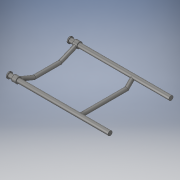
# Autodesk Inventor part: front bar
Saved by Autodesk Inventor 2018 (Build 220112000, 112)
## iProperties
Created: 2018-01-14
Part Number: front bar
Material: Aluminum 6061
Document SubType Name: Modeling
Designer: prakh
Density: 2.7 g/cm^3
Appearance: Anodized - Light Gray
Author: prakh
Autodesk Inventor part; units mm, degrees
ref_plane "XZ Plane" through (0, 0, 0) normal (0, 1, 0) x (-1, 0, 0)
ref_plane "XY Plane" through (0, 0, 0) normal (0, 0, 1) x (1, 0, 0)
sketch "Sketch1" plane through (0, 0, 0) normal (0, 0, 1) x (1, 0, 0)
  circle A0 centre (0, 0) radius 12.7
  dimension "d0" = 25.4
  constraints: 1 centre point, 1 coincident
  measures "d0" diameter of A0
sketch "Sketch2" plane through (0, 0, 0) normal (1, 0, 0) x (0, 1, 0)
  line L0 (0, 88.9) -> (0, -88.9)
  line L1 (0, -88.9) -> (48.2558, -206.375)
  line L2 (0, 88.9) -> (48.2558, 206.375)
  line L3 (48.2558, -206.375) -> (232.1871, -206.375) construction
  point P0 (0, 0)
  dimension "d1" = 88.9
  dimension "d2" = 177.8
  dimension "d3" = 412.75
  dimension "d5" = 127
  dimension "d26" = 112.332
  constraints: 8 end point, 2 vertical alignment, 1 equal length, 1 horizontal, 1 vertical
  measures "d1" distance of point (0, 0) L0.end
  measures "d2" distance of L0.start L0.end
  measures "d3" distance of L1.end L2.end
  measures "d5" distance of L0.start L2.end
  measures "d26" angle of L1 L3
sweep "Sweep1" add profiles "Sketch1" path "Sketch2"
ref_plane "Work Plane1" through (381, 0, 0) normal (1, 0, 0) x (0, 1, 0)
sketch "Sketch3" plane through (0, 0, 0) normal (0, 0, 1) x (1, 0, 0)
  circle A0 centre (381, 0) radius 12.7
  point P0 (0, 0)
  dimension "d9" = 381
  dimension "d10" = 25.4
  constraints: 1 centre point
  measures "d9" distance of point (0, 0) A0.centre
  measures "d10" diameter of A0
sketch "Sketch4" plane through (381, 0, 0) normal (1, 0, 0) x (0, 1, 0)
  line L0 (60.0033, 201.5494) -> (36.5083, 211.2006) projected
  line L1 (48.2558, 206.375) -> (0, 158.75)
  line L2 (0, 158.75) -> (0, -158.75)
  line L3 (0, -158.75) -> (48.2558, -206.375)
  line L4 (36.5083, -211.2006) -> (60.0033, -201.5494) projected
  point P0 (0, 0)
  point P1 (0, 0)
  dimension "d11" = 317.5
  dimension "d13" = 0
  constraints: 6 end point, 2 midpoint, 1 equal length, 1 vertical
  measures "d11" distance of L1.end L2.end
  measures "d13" distance from line of point (0, 0) L2
sweep "Sweep2" add profiles "Sketch3" path "Sketch4" path curves L3 L2 L1
sketch "Sketch5" plane through (0, 0, 0) normal (1, 0, 0) x (0, 1, 0)
  line L0 (39.3348, -215.4141) -> (57.1768, -197.3359) projected
  line L1 (36.5083, -211.2006) -> (60.0033, -201.5494) projected
  line L2 (57.1768, 197.3359) -> (39.3348, 215.4141) projected
  line L3 (60.0033, 201.5494) -> (36.5083, 211.2006) projected
  circle A0 centre (48.2558, 206.375) radius 14.351
  circle A1 centre (48.2558, -206.375) radius 14.351
  point P0 (0, 0)
  dimension "d16" = 28.702
  constraints: 2 centre point, 2 midpoint, 1 equal radius
  measures "d16" diameter of A1
extrude "Extrusion1" add sketch "Sketch5" along normal blind 635 and the other way blind 50.8
sketch "Sketch6" plane through (0, 0, 0) normal (1, 0, 0) x (0, 1, 0)
  circle A0 centre (48.2558, 206.375) radius 14.351 projected
  circle A1 centre (48.2558, -206.375) radius 14.351 projected
  circle A2 centre (48.2558, -206.375) radius 19.812
  circle A3 centre (48.2558, 206.375) radius 19.812
  point P0 (0, 0)
  dimension "d21" = 39.624
  constraints: 2 centre point, 2 coincident, 1 equal radius
  measures "d21" diameter of A2
extrude "Extrusion2" add sketch "Sketch6" along normal mid plane 28.575 contours A0 | A1 | A2 | A3
sketch "Sketch7" plane through (-50.8, 48.2558, 206.375) normal (-1, 0, 0) x (0, 0, 1)
  circle A0 centre (-412.75, 0) radius 14.351 projected
  circle A1 centre (0, 0) radius 14.351 projected
  circle A2 centre (-412.75, 0) radius 19.812 projected
  circle A3 centre (0, 0) radius 19.812 projected
  point P0 (-206.375, -48.2558)
extrude "Extrusion3" add sketch "Sketch7" against normal blind 6.35 contours A0 | A1 | A2 | A3
equation "\"d1\" = 0.5 * d2"
body "Solid1"
